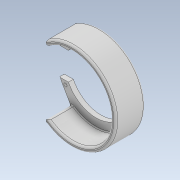
# Autodesk Inventor part: hip_back_motor_protector
Saved by Autodesk Inventor 2020 (Build 240168000, 168)
## iProperties
Created: 2021-01-28
Part Number: hip_back_motor_protector
Material: Generic
Document SubType Name: Modeling
Designer: DELL
Density: 1 g/cm^3
Appearance: Default
Author: DELL
Autodesk Inventor part; units mm, degrees
ref_plane "YZ Plane" through (0, 0, 0) normal (1, 0, 0) x (0, 1, 0)
ref_plane "XZ Plane" through (0, 0, 0) normal (0, 1, 0) x (-1, 0, 0)
ref_plane "XY Plane" through (0, 0, 0) normal (0, 0, 1) x (1, 0, 0)
sketch "Sketch1" plane through (0, 0, 0) normal (0, 0, 1) x (1, 0, 0)
  circle A0 centre (0, 0) radius 31.5
  circle A1 centre (0, 0) radius 40
  circle A2 centre (0, 0) radius 36 construction
  circle A3 centre (0, 0) radius 45
  line L0 (0, 0) -> (-38.9711, 22.5) construction
  line L1 (0, 0) -> (-38.9711, -22.5) construction
  line L2 (0, 0) -> (38.9711, 22.5) construction
  line L3 (0, 0) -> (38.9711, -22.5) construction
  line L4 (-45, 0) -> (45, 0) construction
  line L5 (0, 45) -> (0, -45) construction
  circle A4 centre (-31.1769, 18) radius 1.65
  circle A5 centre (-31.1769, -18) radius 1.65
  circle A6 centre (31.1769, -18) radius 1.65
  circle A7 centre (31.1769, 18) radius 1.65
  line L6 (-34.641, 20) -> (-24.3333, 37.8536)
  line L7 (-34.641, -20) -> (-24.3333, -37.8536)
  line L8 (-28.2179, 14) -> (-37.47, 14)
  line L9 (-28.2179, -14) -> (-37.47, -14)
  dimension "d1" = 90
  dimension "d0" = 80
  dimension "d2" = 63
  dimension "d3" = 72
  dimension "d4" = 30
  dimension "d5" = 30
  dimension "d6" = 3.3
  dimension "d14" = 28
  constraints: 20 end point, 10 point on circle, 7 centre point, 6 point on line, 4 coincident, 4 midpoint, 3 equal radius, 2 horizontal, 2 tangent, 1 vertical, 15 other
  measures "d0" diameter of A1
  measures "d2" diameter of A0
  measures "d3" diameter of A2
  measures "d4" angle of L4 L0
  measures "d5" angle of L4 L1
  measures "d6" diameter of A4
  measures "d14" distance between parallel lines of L9 L8
extrude "Extrusion1" add sketch "Sketch1" along normal blind 5 contours A0 L8 A1 L9 | L6 A3 L7 A1 picked at (-18.8747, -31.7691) picked at (23.161, -34.4452)
extrude "Extrusion2" add sketch "Sketch1" along normal blind 25 from surface at 5 contours L6 A3 L7 A1 picked at (23.161, -34.4452)
fillet "Fillet1" radius 2 7 edges at (-34.641, 20, 17.5) (-34.641, -20, 17.5) (40, 0, 30) (45, 0, 30) (45, 0, 0) (-24.3333, 37.8536, 15) (-24.3333, -37.8536, 15)
fillet "Fillet2" radius 1 3 edges at (-25.3186, 33.0198, 5) (-25.3186, -33.0198, 5) (40, 0, 5)
fillet "Fillet3" radius 1 14 edges at (-36.1801, 17.0587, 5) (-36.1801, -17.0587, 5) (-30.7279, -26.7777, 5) (-26.2241, -34.5785, 5.3262) (-26.2241, 34.5785, 5.3262) (-30.7279, 26.7777, 5) (-36.1801, 17.0587, 0) (-36.1801, -17.0587, 0) (-30.6961, -26.8328, 0) (-25.6074, -35.6466, 0.2094) (-24.2813, -37.822, 1.5354) (-25.6074, 35.6466, 0.2094) (-24.2813, 37.8219, 1.5354) (-30.6961, 26.8328, 0)
body "Solid1"
